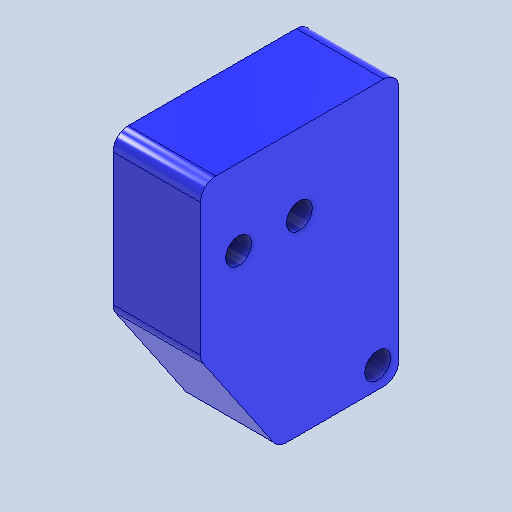
# Autodesk Inventor part: dribl-v1-3DP-l-F-1
Saved by Autodesk Inventor 2025.2 (Build 292293000, 293)
## iProperties
Created: 2025-01-15
Part Number: dribl-v1-3DP-l-F-1
Material: ABS プラスチック
Document SubType Name: Modeling
Designer: haruy
Density: 1.06 g/cm^3
Appearance: 青 - 壁塗料 - 光沢
Author: haruy
Autodesk Inventor part; units mm, degrees
ref_plane "YZ Plane" through (0, 0, 0) normal (1, 0, 0) x (0, 1, 0)
ref_plane "XZ Plane" through (0, 0, 0) normal (0, 1, 0) x (-1, 0, 0)
ref_plane "XY Plane" through (0, 0, 0) normal (0, 0, 1) x (1, 0, 0)
sketch "スケッチ1" plane through (0, 0, 0) normal (1, 0, 0) x (0, 1, 0)
  line L0 (214.6701, 659.5349) -> (214.6701, -648.4651)
  line L1 (214.6701, 627.3349) -> (194.6701, 627.3349)
  line L2 (194.6701, 659.5349) -> (194.6701, -648.4651)
  line L3 (194.6701, 23.5349) -> (214.6701, 23.5349)
  line L4 (194.6701, -648.4651) -> (214.6701, -648.4651)
  line L5 (194.6701, 659.5349) -> (214.6701, 659.5349)
  line L6 (179.6701, 611.4349) -> (207.4701, 611.4349)
  line L7 (207.4701, 611.4349) -> (207.4701, 627.3349)
  line L8 (207.4701, 627.3349) -> (179.6701, 627.3349)
  line L9 (179.6701, 627.3349) -> (179.6701, 611.4349)
  circle A0 centre (182.4701, 614.2349) radius 1.7
  circle A1 centre (204.6701, 624.5349) radius 1.7
  circle A2 centre (204.6701, 632.5349) radius 1.7
  line L10 (179.6701, 77.6349) -> (207.4701, 77.6349)
  line L11 (207.4701, 77.6349) -> (207.4701, 61.7349)
  line L12 (207.4701, 61.7349) -> (179.6701, 61.7349)
  line L13 (179.6701, 61.7349) -> (179.6701, 77.6349)
  circle A3 centre (182.4701, 74.8349) radius 1.5
  circle A4 centre (204.6701, 64.5349) radius 1.5
  circle A5 centre (204.6701, 56.5349) radius 1.5
  line L14 (194.6701, 637.5349) -> (214.6701, 637.5349)
  line L15 (207.4701, 611.4349) -> (214.6701, 611.4349)
  line L16 (214.6701, 611.4349) -> (214.6701, 637.5349)
  line L17 (194.6701, 637.5349) -> (179.6701, 627.3349)
  point P0 (0, 0)
  point P1 (-205.3299, -216.1317)
  dimension "d0" = 672
  dimension "d1" = 27.8
  dimension "d2" = 15.9
  dimension "d3" = 3.4
  dimension "d4" = 3.4
  dimension "d5" = 2.8
  dimension "d6" = 2.8
  dimension "d7" = 2.8
  dimension "d8" = 2.8
  dimension "d9" = 0
  dimension "d10" = 10
  dimension "d11" = 3.4
  dimension "d12" = 8
  dimension "d13" = 10
  dimension "d14" = 27
  dimension "d15" = 27.8
  dimension "d16" = 15.9
  dimension "d17" = 3
  dimension "d18" = 3
  dimension "d19" = 2.8
  dimension "d20" = 2.8
  dimension "d21" = 2.8
  dimension "d22" = 2.8
  dimension "d23" = 10
  dimension "d24" = 560
  dimension "d25" = 3
  dimension "d26" = 8
  dimension "d27" = 10
  dimension "d28" = 5
  constraints: 36 end point, 7 point on line, 6 centre point, 5 perpendicular, 4 horizontal, 4 parallel
  measures "d0" distance between parallel lines of L4 L3
  measures "d1" distance of L8.end L7.end
  measures "d2" distance of L7.end L6.end
  measures "d3" diameter of A0
  measures "d4" diameter of A1
  measures "d5" distance from line of A0.centre L6
  measures "d6" distance from line of A0.centre L9
  measures "d7" distance from line of A1.centre L8
  measures "d8" distance from line of L7 A1.centre
  measures "d9" distance between parallel lines of L1 L8
  measures "d10" distance from line of A1.centre L2
  measures "d11" diameter of A2
  measures "d12" distance of A1.centre A2.centre
  measures "d13" distance from line of L2 A2.centre
  measures "d14" distance from line of A2.centre L5
  measures "d15" distance of L11.end L12.end
  measures "d16" distance of L10.end L11.end
  measures "d17" diameter of A3
  measures "d18" diameter of A4
  measures "d19" distance from line of A3.centre L10
  measures "d20" distance from line of A3.centre L13
  measures "d21" distance from line of A4.centre L12
  measures "d22" distance from line of L11 A4.centre
  measures "d23" distance from line of L0 A4.centre
  measures "d24" distance of A1.centre A4.centre
  measures "d25" diameter of A5
  measures "d26" distance of A5.centre A4.centre
  measures "d27" distance from line of A5.centre L2
  measures "d28" distance from line of A2.centre L14
extrude "押し出し1" add sketch "スケッチ1" against normal blind 11.5 contours L0 L1 L2 L14 | L0 L15 L7 L1 | L2 L8 L17 | L7 L6 L2 L1 | L2 L6 L9 L8
fillet "フィレット1" radius 2 5 edges at (-5.75, 194.6701, 637.5349) (-5.75, 214.6701, 637.5349) (-5.75, 214.6701, 611.4349) (-5.75, 179.6701, 611.4349) (-5.75, 179.6701, 627.3349)
equation "\"d6\" = d5"
equation "\"d7\" = d5"
equation "\"d8\" = d5"
equation "\"d20\" = d19"
equation "\"d21\" = d19"
equation "\"d22\" = d19"
